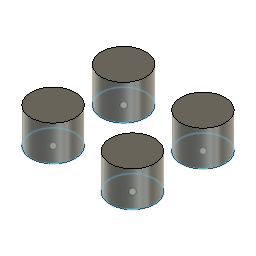
Final Assembly Macropad (Autodesk Fusion 360 archive; units mm, degrees)
design "cyclinders"
part number: 2026-02-26-00-14-27-917
Autodesk Fusion 360 part; units mm, degrees
sketch "Sketch1" plane through (0, 0, 0) normal (0, 0, 1) x (1, 0, 0)
  circle A0 centre (6, 5) radius 2.5
  circle A1 centre (15, 5) radius 2.5
  circle A2 centre (6, 13) radius 2.5
  circle A3 centre (15, 13) radius 2.5
  dimension "d1" = 5
  dimension "d2" = 5
  dimension "d3" = 5
  dimension "d4" = 5
  measures "d1" diameter of A0
  measures "d2" diameter of A1
  measures "d3" diameter of A2
  measures "d4" diameter of A3
extrude "Extrude1" add sketch "Sketch1" along normal blind 4 contours A2 makes body 1
extrude "Extrude2" add sketch "Sketch1" along normal blind 4 separate body contours A0 makes body 2
extrude "Extrude3" add sketch "Sketch1" along normal blind 4 separate body contours A3 makes body 3
extrude "Extrude4" add sketch "Sketch1" along normal blind 4 separate body contours A1 makes body 4

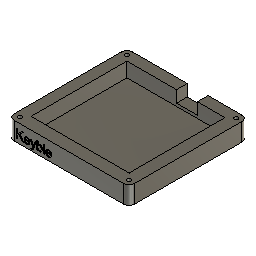
design "Case bottom"
part number: 2026-01-04-20-39-14-527
Autodesk Fusion 360 part; units mm, degrees
sketch "Sketch1" plane through (0, 0, 0) normal (0, 0, 1) x (1, 0, 0)
  line L0 (0, 0) -> (86.91, 0)
  line L1 (86.91, 0) -> (86.91, 85)
  line L2 (86.91, 85) -> (0, 85)
  line L3 (0, 85) -> (0, 0)
  line L4 (97.41, 94.5) -> (-9.5, 94.5)
  line L5 (-9.5, 94.5) -> (-9.5, -10.5)
  line L6 (-9.5, -10.5) -> (97.41, -10.5)
  line L7 (97.41, -10.5) -> (97.41, 94.5)
  circle A0 centre (-4.5, -5.5) radius 1.7
  circle A1 centre (92.41, -5.5) radius 1.7
  circle A2 centre (92.41, 89.5) radius 1.7
  circle A3 centre (-4.5, 89.5) radius 1.7
  circle A4 centre (-4.5, 89.5) radius 3
  circle A5 centre (-4.5, -5.5) radius 3
  circle A6 centre (92.41, -5.5) radius 3
  circle A7 centre (92.41, 89.5) radius 3
  dimension "d1" = 86.91
  dimension "d2" = 85
  dimension "d4" = 106.91
  dimension "d5" = 105
  dimension "d6" = 9.5
  dimension "d7" = 9.5
  dimension "d8" = 3.4
  dimension "d9" = 5
  dimension "d10" = 5
  dimension "d11" = 3.4
  dimension "d12" = 5
  dimension "d13" = 5
  dimension "d14" = 3.4
  dimension "d15" = 5
  dimension "d16" = 5
  dimension "d17" = 3.4
  dimension "d18" = 5
  dimension "d19" = 5
  dimension "d20" = 6
  dimension "d21" = 6
  dimension "d22" = 6
  dimension "d23" = 6
  constraint horizontal L0
  constraint vertical L1
  constraint horizontal L2
  constraint vertical L3
  constraint coincident L0.start L3.end
  constraint horizontal L4
  constraint vertical L5
  constraint horizontal L6
  constraint vertical L7
  constraint concentric A3 A4
  constraint concentric A0 A5
  constraint concentric A1 A6
  constraint concentric A2 A7
  measures "d1" distance of L0.start L0.end
  measures "d2" distance of L0.start L2.end
  measures "d4" distance of L4.start L4.end
  measures "d5" distance of L4.start L6.end
  measures "d6" distance of L2 L4
  measures "d7" distance of L3 L5
  measures "d8" diameter of A0
  measures "d9" distance of L6 A0.centre
  measures "d10" distance of L5 A0.centre
  measures "d11" diameter of A1
  measures "d12" distance of L6 A1.centre
  measures "d13" distance of L7 A1.centre
  measures "d14" diameter of A2
  measures "d15" distance of L4 A2.centre
  measures "d16" distance of L7 A2.centre
  measures "d17" diameter of A3
  measures "d18" distance of L4 A3.centre
  measures "d19" distance of L5 A3.centre
  measures "d20" diameter of A4
  measures "d21" diameter of A5
  measures "d22" diameter of A6
  measures "d23" diameter of A7
sketch "Sketch2" plane through (0, 0, 0) normal (0, 0, 1) x (1, 0, 0)
  line L0 (0, 0) -> (86.91, 0)
  point P0 (0, 85)
  dimension "d3" = 85
  measures "d3" distance of P0 L0
extrude "Extrude1" add sketch "Sketch1" along normal blind 9.9 from surface at 3.1 contours A4 | A5 | A6 | A7 makes body 1 at (94.9699, 91.0643, 9.7) makes body 2 at (95.4063, -5.6495, 9.7) makes body 3 at (-7.2644, 88.3347, 9.7) makes body 4 at (-1.5037, -5.6495, 9.7)
extrude "Extrude2" add sketch "Sketch1" along normal blind 3 separate body contours L0 L1 L2 L3 makes body 5
extrude "Extrude3" add sketch "Sketch1" along normal blind 13 contours L4 L5 L6 L7 bodies 1 2 3 4 5
fillet "Fillet1" radius 5 1 edges at (97.41, -10.5, 6.5) on bodies 1
fillet "Fillet2" radius 5 1 edges at (-9.5, 94.5, 6.5) on bodies 1
fillet "Fillet3" radius 5 1 edges at (97.41, 94.5, 6.5) on bodies 1
fillet "Fillet4" radius 5 1 edges at (-9.5, -10.5, 6.5) on bodies 1
sketch "Sketch3" plane through (0, 0, 13) normal (0, 0, 1) x (-1, 0, 0)
  circle A0 centre (-92.41, 5.5) radius 1.7
  circle A1 centre (4.5, -89.5) radius 1.7
  line L0 (0, 0) -> (0, -85)
  line L1 (0, -85) -> (-86.91, -85)
  line L2 (-86.91, -85) -> (-86.91, 0)
  line L3 (-86.91, 0) -> (0, 0)
  arc A2 (9.5, 5.5) -> (4.5, 10.5) centre (4.5, 5.5) ccw
  line L4 (4.5, 10.5) -> (-92.41, 10.5)
  arc A3 (-92.41, 10.5) -> (-97.41, 5.5) centre (-92.41, 5.5) ccw
  line L5 (-97.41, 5.5) -> (-97.41, -89.5)
  arc A4 (-97.41, -89.5) -> (-92.41, -94.5) centre (-92.41, -89.5) ccw
  line L6 (-92.41, -94.5) -> (4.5, -94.5)
  arc A5 (4.5, -94.5) -> (9.5, -89.5) centre (4.5, -89.5) ccw
  line L7 (9.5, -89.5) -> (9.5, 5.5)
  circle A6 centre (-92.41, -89.5) radius 1.7
  circle A7 centre (4.5, 5.5) radius 1.7
  dimension "d39" = 105
  dimension "d40" = 96.91
  dimension "d41" = 86.91
  dimension "d42" = 85
  measures "d39" distance of A2.end L6.end
  measures "d40" distance of A2.end L4.end
  measures "d41" distance of L0.end L1.end
  measures "d42" distance of L1.end L2.end
sketch "Sketch4" plane through (0, 0, 13) normal (0, 0, 1) x (-1, 0, 0)
  line L0 (-97.41, -94.5) -> (9.5, -94.5)
  line L1 (-43.963, -94.5) -> (-62.463, -94.5)
  line L2 (-62.463, -94.5) -> (-62.463, -85)
  line L3 (-62.463, -85) -> (-43.963, -85)
  line L4 (-43.963, -85) -> (-43.963, -94.5)
  point P0 (-86.91, -85)
  point P1 (0, -85)
  dimension "d43" = 86.91
  dimension "d44" = 9.5
  dimension "d45" = 18.5
  dimension "d47" = 24.447
  constraint horizontal L1
  constraint vertical L2
  constraint horizontal L3
  constraint vertical L4
  constraint coincident L0 L1.start
  measures "d43" distance of P0 P1
  measures "d44" distance of P0 L0
  measures "d45" distance of L1.start L1.end
  measures "d47" distance of P0 L2.end
extrude "Extrude4" cut sketch "Sketch4" against normal blind 7.5 bodies 1
sketch "Sketch5" plane through (0, -10.5, 0) normal (0, -1, 0) x (1, 0, 0)
  line L0 (-4.5, 13) -> (-4.5, 0)
  line L1 (-4.5, 0) -> (92.41, 0)
  line L2 (92.41, 0) -> (92.41, 13)
  line L3 (92.41, 13) -> (-4.5, 13)
  line L4 (-2.4411, 0.2561) -> (29.6899, -0.0005) construction
  line L5 (29.6899, -0.0005) -> (29.7735, 10.4665) construction
  line L6 (29.7735, 10.4665) -> (-2.3575, 10.7231) construction
  line L7 (-2.3575, 10.7231) -> (-2.4411, 0.2561) construction
  line L8 (-4.5, 13) -> (92.41, 13)
  line L9 (-9.5, 0) -> (97.41, 0)
  dimension "d50" = 7.5
  text T0 "Keybie" font "Arial" height 7.5 align left top in box 32.132 x 10.4673 at (-2.4411, 0.2561) x (0.999968, -0.007986) y (0.007986, 0.999968) spacing 1 kerned
extrude "Extrude5" cut sketch "Sketch5" against normal blind 0.2 text T0 bodies 1
move_face "MoveFace1" by (0, 0, 2.8) 1 faces at (58.2733, -7, 13) on bodies 1
move_face "MoveFace2" by (0, 0, 0.07) 1 faces at (29.3087, 90.3931, 15.8) on bodies 1
equation "d51 = 'Keybie'"
